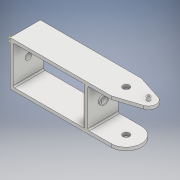
# Autodesk Inventor part: Right forearm
Saved by Autodesk Inventor 2018 (Build 220112000, 112)
## iProperties
Created: 2018-02-08
Part Number: Right forearm
Material: Plastique ABS
Document SubType Name: Modeling
Designer: Thomas
Density: 1.06 g/cm^3
Appearance: Lisse - Blanc
Mass: 115.536 g
Surface Area: 492.913 cm^2
Volume: 108.996 cm^3
Author: Thomas
Autodesk Inventor part; units mm, degrees
ref_plane "YZ Plane" through (0, 0, 0) normal (1, 0, 0) x (0, 1, 0)
ref_plane "XZ Plane" through (0, 0, 0) normal (0, 1, 0) x (-1, 0, 0)
ref_plane "XY Plane" through (0, 0, 0) normal (0, 0, 1) x (1, 0, 0)
sketch "Esquisse1" plane through (0, 0, 0) normal (0, 0, 1) x (1, 0, 0)
  point P0 (0, 0)
sketch "Esquisse2" plane through (0, 0, 0) normal (0, 0, 1) x (1, 0, 0)
  line L0 (0, 0) -> (156, 0)
  line L1 (0, 46.8) -> (0, 0)
  line L2 (194.0737, 12.2634) -> (156, 0)
  arc A0 (194.0737, 12.2634) -> (194.0737, 34.5366) centre (190.4867, 23.4) ccw
  line L3 (0, 46.8) -> (156, 46.8)
  line L4 (156, 46.8) -> (194.0737, 34.5366)
  dimension "d0" = 156
  dimension "d1" = 46.8
  dimension "d2" = 11.7
  dimension "d4" = 40
  dimension "d6" = 40
  constraints: 10 end point, 2 horizontal, 2 point on circle, 1 centre point, 1 tangent
  measures "d0" distance of L3.end L1.start
  measures "d1" distance of L1.start L0.start
  measures "d2" radius of A0
  measures "d4" distance of L3.end L4.end
  measures "d6" distance of L2.start L0.end
extrude "Extrusion1" add sketch "Esquisse2" along normal blind 5
sketch "Esquisse3" plane through (0, 0, 5) normal (0, 0, 1) x (1, 0, 0)
  line L0 (194.0737, 34.5366) -> (156, 46.8) projected
  line L1 (156, 46.8) -> (156, 0)
  circle A0 centre (156, 23.4) radius 5
  point P0 (0, 0)
  dimension "d11" = 23.4
  dimension "d12" = 10
  constraints: 2 end point, 1 centre point, 1 coincident, 1 midpoint, 1 vertical
  measures "d11" distance of L1.end point (156, 23.4)
  measures "d12" diameter of A0
extrude "Extrusion2" cut sketch "Esquisse3" against normal blind 5
sketch "Esquisse4" plane through (0, 0, 5) normal (0, 0, 1) x (1, 0, 0)
  point P0 (0, 0)
sketch "Esquisse5" plane through (0, 0, 5) normal (0, 0, 1) x (1, 0, 0)
  arc A0 (194.0737, 12.2634) -> (194.0737, 34.5366) centre (190.4867, 23.4) ccw projected
  circle A1 centre (190.4867, 23.4) radius 3
  point P0 (0, 0)
  point P1 (194.0737, 12.2634)
  dimension "d17" = 6
  constraints: 3 coincident, 1 centre point
  measures "d17" diameter of A1
extrude "Extrusion3" add sketch "Esquisse5" along normal blind 5
sketch "Esquisse6" plane through (190.4867, 23.4, 10) normal (0, 0, 1) x (1, 0, 0)
  circle A0 centre (0, 0) radius 1.5
  point P0 (-190.4867, -23.4)
  dimension "d20" = 3
  constraints: 1 centre point
  measures "d20" diameter of A0
extrude "Extrusion4" cut sketch "Esquisse6" against normal blind 5
sketch "Esquisse7" plane through (0, 0, 0) normal (-1, 0, 0) x (0, 0, 1)
  line L0 (0, 0) -> (-63.96, 0)
  line L1 (-63.96, 0) -> (-63.96, 46.8)
  line L2 (-63.96, 46.8) -> (0, 46.8)
  line L3 (0, 46.8) -> (0, 0)
  dimension "d23" = 63.96
  dimension "d24" = 46.8
  constraints: 8 end point, 2 parallel, 1 horizontal, 1 perpendicular
  measures "d23" distance of L1.end L2.end
  measures "d24" distance of L2.end L0.start
extrude "Extrusion5" add sketch "Esquisse7" against normal blind 5
sketch "Esquisse8" plane through (0, 0, 5) normal (-1, 0, 0) x (0, 0, 1)
  line L0 (-68.96, 46.8) -> (0, 46.8) projected
  line L1 (-68.96, 46.8) -> (0, 0)
  line L2 (0, 46.8) -> (-68.96, 0)
  circle A0 centre (-34.48, 23.4) radius 7
  point P0 (-5, 0)
  dimension "d27" = 14
  constraints: 4 end point, 1 centre point, 1 coincident, 1 midpoint
  measures "d27" diameter of A0
extrude "Extrusion6" add sketch "Esquisse8" along normal blind 2 contours A0 L2 L1 | L1 L2 A0 | A0 L1 L2 | L1 A0 L2
sketch "Esquisse9" plane through (-2, 23.4, -29.48) normal (-1, 0, 0) x (0, 0, 1)
  circle A0 centre (0, 0) radius 5
  point P0 (29.48, -23.4)
  dimension "d30" = 10
  constraints: 1 centre point
  measures "d30" diameter of A0
extrude "Extrusion7" cut sketch "Esquisse9" against normal blind 7
sketch "Esquisse10" plane through (0, 0, -63.96) normal (0, 0, -1) x (-1, 0, 0)
  line L0 (-5, 0) -> (-5, 46.8) projected
  line L1 (-5, 46.8) -> (-156, 46.8)
  line L2 (-156, 0) -> (-5, 0)
  line L3 (-5, 0) -> (-5, 46.8)
  arc A0 (-156, 46.8) -> (-156, 0) centre (-156, 23.4) ccw
  point P0 (0, 0)
  dimension "d33" = 151
  constraints: 6 end point, 2 point on circle, 1 centre point, 1 coincident, 1 horizontal, 1 parallel
  measures "d33" distance of L2.start L2.end
extrude "Extrusion8" add sketch "Esquisse10" against normal blind 5
sketch "Esquisse11" plane through (0, 0, -63.96) normal (0, 0, -1) x (-1, 0, 0)
  arc A0 (-156, 46.8) -> (-156, 0) centre (-156, 23.4) ccw projected
  circle A1 centre (-156, 23.4) radius 5
  point P0 (0, 0)
  dimension "d36" = 10
  constraints: 2 coincident, 1 centre point
  measures "d36" diameter of A1
extrude "Extrusion9" cut sketch "Esquisse11" against normal blind 5
ref_plane "Plan de construction1" through (115.24, 0, 0) normal (1, 0, 0) x (0, 0, -1)
sketch "Esquisse12" plane through (115.24, 0, 0) normal (1, 0, 0) x (0, 0, -1)
  line L0 (0, 0) -> (0, 13)
  line L1 (0, 0) -> (0, 46.8) projected
  line L2 (0, 13) -> (2, 13)
  line L3 (0, 0) -> (58.96, 0)
  line L4 (58.96, 0) -> (58.96, 46.8)
  line L5 (12, 23) -> (12, 31.8)
  line L6 (27, 46.8) -> (58.96, 46.8)
  arc A0 (2, 13) -> (12, 23) centre (2, 23) ccw
  arc A1 (27, 46.8) -> (12, 31.8) centre (27, 31.8) ccw
  point P0 (12, 13)
  dimension "d40" = 13
  dimension "d41" = 12
  dimension "d42" = 46.8
  dimension "d44" = 10
  dimension "d45" = 15
  constraints: 12 end point, 4 point on circle, 4 tangent, 3 point on line, 2 centre point, 2 horizontal, 2 vertical, 1 perpendicular
  measures "d40" distance of L0.start L0.end
  measures "d41" distance of L0.end point (12, 13)
  measures "d42" distance of L3.end L4.end
  measures "d44" radius of A0
  measures "d45" radius of A1
extrude "Extrusion10" add sketch "Esquisse12" along normal blind 5
fillet "Congé1" radius 2 4 edges at (120.24, 6.5, 0) (120.24, 23.4, -58.96) (115.24, 23.4, -58.96) (115.24, 6.5, 0)
fillet "Congé2" radius 2 2 edges at (5, 23.4, 0) (5, 23.4, -58.96)
sketch "Esquisse13" plane through (120.24, 0, 0) normal (1, 0, 0) x (0, 0, -1)
  line L0 (63.96, 46.8) -> (-5, 46.8) projected
  line L1 (0, 46.8) -> (58.706, 0)
  line L2 (58.706, 46.8) -> (0, 0)
  circle A0 centre (29.353, 23.4) radius 7
  dimension "d51" = 14
  constraints: 4 end point, 2 point on line, 1 centre point, 1 coincident, 1 midpoint
  measures "d51" diameter of A0
extrude "Extrusion11" add sketch "Esquisse13" along normal blind 2 contours A0 L1 L2 | L2 L1 A0 | L1 L2 A0 | L1 A0 L2
sketch "Esquisse14" plane through (122.24, 23.4, -29.353) normal (1, 0, 0) x (0, 0, -1)
  circle A0 centre (0, 0) radius 5
  point P0 (-29.353, -23.4)
  dimension "d54" = 10
  constraints: 1 centre point
  measures "d54" diameter of A0
extrude "Extrusion12" cut sketch "Esquisse14" against normal blind 7
